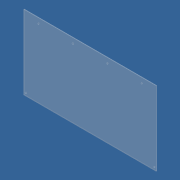
# Autodesk Inventor part: GE-12051
Saved by Autodesk Inventor 2012 (Build 160160000, 160)
## iProperties
Created: 2011-05-23
Part Number: GE-12051
Document SubType Name: Modeling
Designer: dfoster
Density: 1 g/cm^3
Description: Inbound Plastic
Material: Default
Title: Inbound Plastic
Author: dfoster
Autodesk Inventor part; units mm, degrees
ref_plane "YZ Plane" through (0, 0, 0) normal (1, 0, 0) x (0, 1, 0)
ref_plane "XZ Plane" through (0, 0, 0) normal (0, 1, 0) x (-1, 0, 0)
ref_plane "XY Plane" through (0, 0, 0) normal (0, 0, 1) x (1, 0, 0)
sketch "Sketch1" plane through (0, 0, 0) normal (0, 0, 1) x (1, 0, 0)
  line L0 (0, 0) -> (1270, 0)
  line L1 (1270, 0) -> (1270, 711.2)
  line L2 (1270, 711.2) -> (0, 711.2)
  line L3 (0, 711.2) -> (0, 0)
  dimension "d0" = 1270
  dimension "d1" = 711.2
  constraints: 8 end point, 2 parallel, 1 horizontal, 1 perpendicular
  measures "d0" distance of L1.end L2.end
  measures "d1" distance of L2.end L0.start
extrude "Extrusion1" add sketch "Sketch1" along normal blind 6.35
hole "Hole1" at (139.7, 660.4, 6.35) direction (0, 0, -1) diameter 12.7 end through all
pattern_linear "Rectangular Pattern1" count 4 spacing 330.2 along (1, 0, 0) of "Hole1"
hole "Hole2" at (19.05, 25.4, 6.35) direction (0, 0, -1) diameter 12.7 end through all
pattern_linear "Rectangular Pattern2" count 2 spacing 1231.9 along (1, 0, 0) of "Hole2"
body "Solid1"
